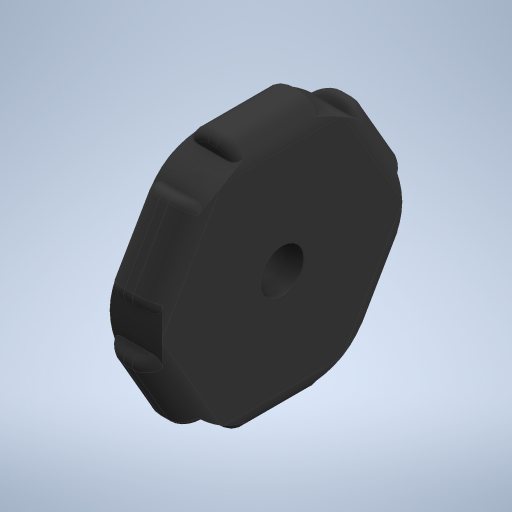
# Autodesk Inventor part: roue
Saved by Autodesk Inventor 2024.1 (Build 281209000, 209)
## iProperties
Created: 2024-04-29
Part Number: roue
Material: Générique
Document SubType Name: Modeling
Designer: chass
Density: 1 g/cm^3
Appearance: Par défaut
Author: chass
Autodesk Inventor part; units mm, degrees
ref_plane "YZ Plane" through (0, 0, 0) normal (1, 0, 0) x (0, 1, 0)
ref_plane "XZ Plane" through (0, 0, 0) normal (0, 1, 0) x (-1, 0, 0)
ref_plane "XY Plane" through (0, 0, 0) normal (0, 0, 1) x (1, 0, 0)
sketch "Esquisse1" plane through (0, 0, 0) normal (1, 0, 0) x (0, 1, 0)
  circle A0 centre (0, 0) radius 27.5
  line L0 (29, 10) -> (24, 10)
  line L1 (24, 10) -> (24, -10)
  line L2 (24, -10) -> (29, -10)
  line L3 (29, -10) -> (29, 10)
  line L4 (3.3397, 25.7846) -> (20.6603, 15.7846)
  line L5 (20.6603, 15.7846) -> (23.1603, 20.1147)
  line L6 (23.1603, 20.1147) -> (5.8397, 30.1147)
  line L7 (5.8397, 30.1147) -> (3.3397, 25.7846)
  line L8 (-20.6603, 15.7846) -> (-3.3397, 25.7846)
  line L9 (-3.3397, 25.7846) -> (-5.8397, 30.1147)
  line L10 (-5.8397, 30.1147) -> (-23.1603, 20.1147)
  line L11 (-23.1603, 20.1147) -> (-20.6603, 15.7846)
  line L12 (-24, -10) -> (-24, 10)
  line L13 (-24, 10) -> (-29, 10)
  line L14 (-29, 10) -> (-29, -10)
  line L15 (-29, -10) -> (-24, -10)
  line L16 (-3.3397, -25.7846) -> (-20.6603, -15.7846)
  line L17 (-20.6603, -15.7846) -> (-23.1603, -20.1147)
  line L18 (-23.1603, -20.1147) -> (-5.8397, -30.1147)
  line L19 (-5.8397, -30.1147) -> (-3.3397, -25.7846)
  line L20 (20.6603, -15.7846) -> (3.3397, -25.7846)
  line L21 (3.3397, -25.7846) -> (5.8397, -30.1147)
  line L22 (5.8397, -30.1147) -> (23.1603, -20.1147)
  line L23 (23.1603, -20.1147) -> (20.6603, -15.7846)
  point P0 (4.1484, 27.1853)
  point P1 (-4.1484, 27.1853)
  point P2 (-21.4689, 17.1853)
  point P3 (-25.6174, 10)
  point P4 (-25.6174, -10)
  point P5 (-21.4689, -17.1853)
  point P6 (-4.1484, -27.1853)
  point P7 (4.1484, -27.1853)
  point P8 (21.4689, -17.1853)
  point P9 (25.6174, -10)
  point P10 (25.6174, 10)
  point P11 (21.4689, 17.1853)
  dimension "d0" = 55
  dimension "d3" = 360
  constraints: 48 end point, 2 parallel, 1 centre point, 1 coincident, 1 horizontal, 1 perpendicular, 49 other
  measures "d0" diameter of A0
extrude "Extrusion1" add sketch "Esquisse1" along normal blind 12
fillet "Congé1" radius 5 12 edges at (0, 14.5, 25.1147) (12, 14.5, 25.1147) (0, 29, 0) (12, 29, 0) (0, 14.5, -25.1147) (12, 14.5, -25.1147) (0, -14.5, -25.1147) (12, -14.5, -25.1147) (0, -29, 0) (12, -29, 0) (0, -14.5, 25.1147) (12, -14.5, 25.1147)
fillet "Congé2" radius 2 36 edges at (9.908, 28.0674, 10) (2.092, 28.0674, 10) (6, 29, 10) (6, 23.1603, 20.1147) (2.092, 22.6939, 19.307) (9.908, 22.6939, 19.307) (6, 29, -10) (2.092, 28.0674, -10) (9.908, 28.0674, -10) (6, 23.1603, -20.1147) (2.092, 22.6939, -19.307) (9.908, 22.6939, -19.307) (6, 5.8397, -30.1147) (2.092, 5.3734, -29.307) (9.908, 5.3734, -29.307) (6, -5.8397, -30.1147) (2.092, -5.3734, -29.307) (9.908, -5.3734, -29.307) (6, -23.1603, -20.1147) (2.092, -22.6939, -19.307) (9.908, -22.6939, -19.307) (6, -29, -10) (2.092, -28.0674, -10) (9.908, -28.0674, -10) (6, -29, 10) (2.092, -28.0674, 10) (9.908, -28.0674, 10) (6, -23.1603, 20.1147) (2.092, -22.6939, 19.307) (9.908, -22.6939, 19.307) (6, -5.8397, 30.1147) (2.092, -5.3734, 29.307) (9.908, -5.3734, 29.307) (6, 5.8397, 30.1147) (2.092, 5.3734, 29.307) (9.908, 5.3734, 29.307)
sketch "Esquisse2" plane through (12, 0, 0) normal (1, 0, 0) x (0, 0, -1)
  circle A0 centre (0, 0) radius 5
  dimension "d9" = 10
  constraints: 1 centre point, 1 coincident
  measures "d9" diameter of A0
extrude "Extrusion2" cut sketch "Esquisse2" against normal blind 12
